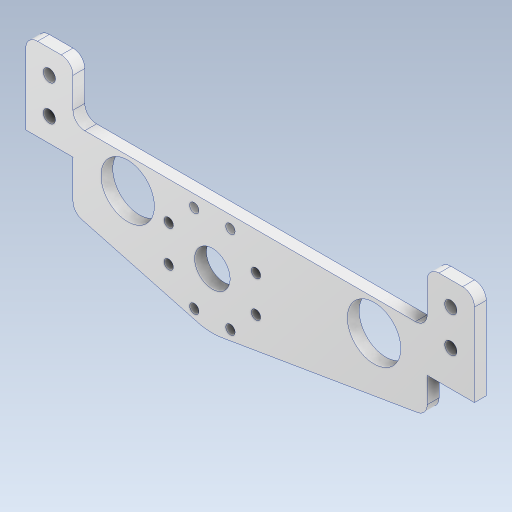
# Autodesk Inventor part: INDX_004_shufflePlate
Saved by Autodesk Inventor 2024 (Build 280153000, 153)
## iProperties
Created: 2024-08-08
Part Number: INDX_004_shufflePlate
Material: Aluminum 6061
Document SubType Name: Modeling
Designer: Oscar
Density: 2.7 g/cm^3
Appearance: Aluminum - Flat
Author: Oscar
Autodesk Inventor part; units mm, degrees
ref_plane "YZ Plane" through (0, 0, 0) normal (1, 0, 0) x (0, 1, 0)
ref_plane "XZ Plane" through (0, 0, 0) normal (0, 1, 0) x (-1, 0, 0)
ref_plane "XY Plane" through (0, 0, 0) normal (0, 0, 1) x (1, 0, 0)
sketch "Sketch1" plane through (0, 0, 0) normal (0, 0, 1) x (1, 0, 0)
  line L0 (0, 0) -> (-812.8, 0) construction
  line L1 (-812.8, 0) -> (-812.8, 50.8) construction
  line L2 (-812.8, 50.8) -> (0, 50.8) construction
  line L3 (0, 50.8) -> (0, 0) construction
  circle A0 centre (-279.4, 50.8) radius 25.4 construction
  circle A1 centre (-279.4, 200.025) radius 25.4 construction
  line L4 (-241.3, 50.8) -> (-215.9, 50.8) construction
  line L5 (-215.9, 50.8) -> (-215.9, 0) construction
  line L6 (-215.9, 0) -> (-241.3, 0) construction
  line L7 (-241.3, 0) -> (-241.3, 50.8) construction
  line L8 (-355.6, 0) -> (-330.2, 0) construction
  line L9 (-330.2, 0) -> (-330.2, 762) construction
  line L10 (-330.2, 762) -> (-355.6, 762) construction
  line L11 (-355.6, 762) -> (-355.6, 0) construction
  line L12 (-241.3, 50.8) -> (-215.9, 50.8) construction
  line L13 (0, 50.8) -> (-25.4, 50.8) construction
  line L14 (-25.4, 50.8) -> (-25.4, 0) construction
  line L15 (-25.4, 0) -> (0, 0) construction
  line L16 (0, 0) -> (0, 50.8) construction
  circle A2 centre (-186.4868, 56.1467) radius 14.351
  circle A3 centre (-53.975, 56.1467) radius 14.351
  circle A4 centre (-186.4868, 56.1467) radius 17.5133 construction
  line L17 (-279.4, 76.2) -> (3.6052, 76.2) construction
  circle A5 centre (-186.4868, 56.1467) radius 20.0533 construction
  line L18 (-215.9, 50.8) -> (-241.3, 50.8) construction
  line L19 (-241.3, 50.8) -> (-241.3, 101.6) construction
  line L20 (-215.9, 101.6) -> (-215.9, 50.8) construction
  circle A6 centre (-53.975, 56.1467) radius 20.0533 construction
  line L21 (-25.4, 50.8) -> (0, 50.8)
  circle A7 centre (-228.6, 69.85) radius 3.2639
  circle A8 centre (-12.7, 69.85) radius 3.2639
  circle A9 centre (-186.4868, 56.1467) radius 16.51 construction
  circle A10 centre (-53.975, 56.1467) radius 16.51 construction
  line L22 (-215.9, 72.6567) -> (-25.4, 72.6567)
  circle A11 centre (-12.7, 88.9) radius 3.2639
  line L23 (0, 50.8) -> (0, 101.6)
  line L24 (0, 101.6) -> (-25.4, 101.6)
  line L25 (-25.4, 101.6) -> (-25.4, 72.6567)
  line L26 (-215.9, 50.8) -> (-241.3, 50.8)
  line L27 (-241.3, 101.6) -> (-241.3, 50.8)
  line L28 (-241.3, 101.6) -> (-215.9, 101.6)
  line L29 (-215.9, 101.6) -> (-215.9, 72.6567)
  circle A12 centre (-140.9402, 42.672) radius 29.972 construction
  circle A13 centre (-140.9402, 42.672) radius 25.4 construction
  circle A14 centre (-140.9402, 42.672) radius 9.525
  circle A15 centre (-131.22, 66.1385) radius 2.4892
  circle A16 centre (-150.6604, 66.1385) radius 2.4892
  circle A17 centre (-164.4067, 52.3922) radius 2.4892
  circle A18 centre (-164.4067, 32.9518) radius 2.4892
  circle A19 centre (-150.6604, 19.2055) radius 2.4892
  circle A20 centre (-131.22, 19.2055) radius 2.4892
  circle A21 centre (-140.9402, 42.672) radius 10.16 construction
  line L30 (-140.9402, 0) -> (-140.9402, 12.7) construction
  line L31 (-25.4, 50.8) -> (-25.4, 31.75)
  line L32 (-25.4, 31.75) -> (-135.9591, 13.1168)
  line L33 (-215.9, 50.8) -> (-215.9, 31.75)
  line L34 (-215.9, 31.75) -> (-148.7063, 13.7236)
  arc A22 (-148.7063, 13.7236) -> (-135.9591, 13.1168) centre (-140.9402, 42.672) ccw
  circle A23 centre (-228.6, 88.9) radius 3.2639
  circle A24 centre (-117.4737, 32.9518) radius 2.4892
  circle A25 centre (-117.4737, 52.3922) radius 2.4892
  line L35 (-241.3, 50.8) -> (-215.9, 50.8)
  line L36 (-215.9, 50.8) -> (-215.9, 57.15)
  line L37 (-215.9, 57.15) -> (-241.3, 57.15)
  line L38 (-241.3, 57.15) -> (-241.3, 50.8)
  point P0 (0, 25.4)
  point P1 (-171.4526, 62.9697)
  point P2 (-186.4868, 72.6567)
  dimension "d2" = 50.8
  dimension "d59" = 50.8
  dimension "d0" = 812.8
  dimension "d1" = 50.8
  dimension "d4" = 279.4
  dimension "d5" = 25.4
  dimension "d6" = 215.9
  dimension "d7" = 25.4
  dimension "d8" = 762
  dimension "d9" = 330.2
  dimension "d13" = 25.4
  dimension "d14" = 50.8
  dimension "d15" = 28.702
  dimension "d16" = 35.0266
  dimension "d17" = 2.54
  dimension "d26" = 132.5118
  dimension "d34" = 28.575
  dimension "d38" = 6.5278
  dimension "d39" = 19.05
  dimension "d40" = 12.7
  dimension "d47" = 33.02
  dimension "d48" = 19.05
  dimension "d50" = 19.05
  dimension "d51" = 25.4
  dimension "d52" = 50.8
  dimension "d54" = 12.7
  dimension "d55" = 50.8
  dimension "d58" = 59.944
  dimension "d60" = 19.05
  dimension "d61" = 4.9784
  dimension "d64" = 360
  dimension "d66" = 20.32
  dimension "d68" = 12.7
  dimension "d69" = 47.498
  dimension "d70" = 25.4
  dimension "d71" = 19.05
  dimension "d72" = 19.05
  dimension "d73" = 19.05
  dimension "d75" = 25.4
  dimension "d76" = 6.35
  constraints: 78 end point, 24 centre point, 12 equal length, 11 horizontal, 11 point on line, 10 perpendicular, 7 coincident, 7 point on circle, 6 equal radius, 5 vertical alignment, 4 tangent, 2 vertical, 1 concentric, 1 horizontal alignment, 1 midpoint, 23 other
  measures "d0" distance of L1.end L2.end
  measures "d1" distance between parallel lines of L0 L2
  measures "d4" distance from line of L3 point (-279.4, 50.8)
  measures "d5" distance of L5.end L6.end
  measures "d6" distance between parallel lines of L3 L5
  measures "d7" distance of L10.end L9.end
  measures "d8" distance of L9.end L8.end
  measures "d9" distance from line of point (0, 25.4) L9
  measures "d13" distance of L15.end L14.end
  measures "d14" distance of L14.end L13.end
  measures "d15" diameter of A2
  measures "d16" diameter of A4
  measures "d17" radial gap between concentric circles of A4 A5
  measures "d26" distance of A3.centre A2.centre
  measures "d34" distance from line of L14 A3.centre
  measures "d38" diameter of A7
  measures "d39" distance from line of L2 A7.centre
  measures "d40" distance from line of L19 A7.centre
  measures "d47" diameter of A10
  measures "d48" distance from line of A8.centre L2
  measures "d50" distance of A11.centre A8.centre
  measures "d51" distance of L23.end L24.end
  measures "d52" distance of L2.end L23.end
  measures "d54" distance from line of L23 A8.centre
  measures "d55" distance between parallel lines of L4 L28
  measures "d58" diameter of A12
  measures "d60" diameter of A14
  measures "d61" diameter of A15
  measures "d66" diameter of A21
  measures "d68" distance of L30.start L30.end
  measures "d69" distance of A12.centre A2.centre
  measures "d70" distance from line of L4.end L19
  measures "d71" distance of L13.end L31.end
  measures "d72" distance of L4.end L33.end
  measures "d73" distance of A7.centre A23.centre
  measures "d75" distance of L37.end L36.end
  measures "d76" distance of L36.end L35.end
extrude "Extrusion1" add sketch "Sketch1" along normal blind 6.35 contours L31 L32 A22 L34 L33 L36 L37 L27 L28 L29 L22 L25 L24 L23 L21
fillet "Fillet2" radius 6.35 8 edges at (-215.9, 72.6567, 3.175) (-25.4, 72.6567, 3.175) (-241.3, 101.6, 3.175) (-215.9, 101.6, 3.175) (0, 101.6, 3.175) (-25.4, 101.6, 3.175) (-25.4, 31.75, 3.175) (-215.9, 31.75, 3.175)
body "Solid1"
